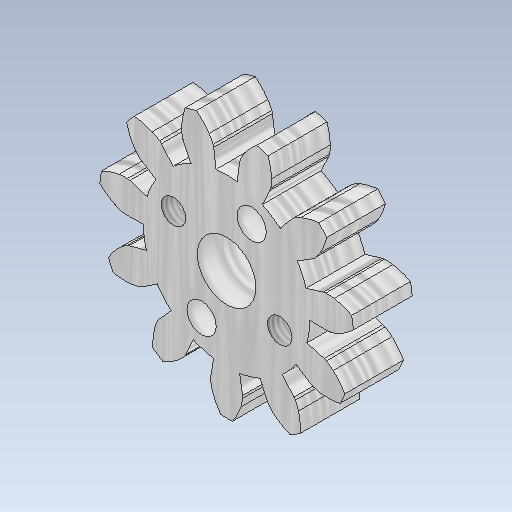
# Autodesk Inventor part: ｍ2歯数11ギア6td6
Saved by Autodesk Inventor 2020.2 (Build 242310000, 310)
## iProperties
Created: 2020-02-29
Part Number: ｍ2歯数11ギア6td6
Material: アルミニウム 7075
Document SubType Name: Modeling
Designer: aoyam
Density: 2.81 g/cm^3
Appearance: サテン - ブラシ仕上げ 重厚
Mass: 5.22906 g
Surface Area: 18.0274 cm^2
Volume: 1.86088 cm^3
Author: aoyam
Autodesk Inventor part; units mm, degrees
ref_plane "YZ Plane" through (0, 0, 0) normal (1, 0, 0) x (0, 1, 0)
ref_plane "XZ Plane" through (0, 0, 0) normal (0, 1, 0) x (-1, 0, 0)
ref_plane "XY Plane" through (0, 0, 0) normal (0, 0, 1) x (1, 0, 0)
sketch "スケッチ1" plane through (0, 0, 0) normal (0, 0, 1) x (1, 0, 0)
  arc A0 (-0.8026, 11.5515) -> (-0.8708, 11.3096) centre (0.3876, 11.0851) ccw
  arc A1 (-0.4025, 12.3114) -> (-0.8026, 11.5515) centre (2.526, 10.2842) ccw
  arc A2 (0.8885, 13.6879) -> (-0.4025, 12.3114) centre (4.8143, 8.7121) ccw
  arc A3 (-3.5076, 11.3096) -> (-3.5759, 11.5515) centre (-4.7661, 11.0851) ccw
  arc A4 (-3.5759, 11.5515) -> (-3.976, 12.3114) centre (-6.9045, 10.2842) ccw
  arc A5 (-3.976, 12.3114) -> (-5.267, 13.6879) centre (-9.1928, 8.7121) ccw
  arc A6 (-1.1051, 9.488) -> (-3.2734, 9.488) centre (-2.1892, 1.0574) ccw
  arc A7 (-5.267, 13.6879) -> (-6.4286, 13.3468) centre (-2.1892, 1.0574) ccw
  line L0 (-1.1051, 9.488) -> (-0.8708, 11.3096)
  line L1 (-3.2734, 9.488) -> (-3.5076, 11.3096)
  arc A8 (-6.6962, 10.6353) -> (-6.6229, 10.3949) centre (-5.4428, 10.8864) ccw
  arc A9 (-5.8351, 8.7358) -> (-7.6592, 7.5635) centre (-2.1892, 1.0574) ccw
  line L2 (-5.8351, 8.7358) -> (-6.6229, 10.3949)
  arc A10 (-6.7705, 11.4908) -> (-6.6962, 10.6353) centre (-3.2109, 11.3688) ccw
  arc A11 (-6.4286, 13.3468) -> (-6.7705, 11.4908) centre (-0.4359, 11.2834) ccw
  line L3 (-7.6592, 7.5635) -> (-8.8411, 8.9693)
  arc A12 (-8.8411, 8.9693) -> (-9.0293, 9.1359) centre (-9.7784, 8.1001) ccw
  arc A13 (-9.0293, 9.1359) -> (-9.7767, 9.5589) centre (-11.1444, 6.2702) ccw
  arc A14 (-11.6069, 10.0189) -> (-12.3997, 9.1039) centre (-2.1892, 1.0574) ccw
  arc A15 (-9.7767, 9.5589) -> (-11.6069, 10.0189) centre (-12.2195, 3.7106) ccw
  arc A16 (-11.159, 6.6782) -> (-10.9673, 6.5156) centre (-10.2402, 7.5671) ccw
  arc A17 (-9.4076, 5.5458) -> (-10.3083, 3.5734) centre (-2.1892, 1.0574) ccw
  line L4 (-9.4076, 5.5458) -> (-10.9673, 6.5156)
  arc A18 (-11.6839, 7.3577) -> (-11.159, 6.6782) centre (-8.6234, 9.1796) ccw
  arc A19 (-12.3997, 9.1039) -> (-11.6839, 7.3577) centre (-6.2428, 10.608) ccw
  line L5 (-10.3083, 3.5734) -> (-12.0626, 4.1171)
  arc A20 (-12.0626, 4.1171) -> (-12.311, 4.1555) centre (-12.3812, 2.8791) ccw
  arc A21 (-12.311, 4.1555) -> (-13.1684, 4.1072) centre (-12.541, 0.6012) ccw
  arc A22 (-14.9568, 3.5047) -> (-15.1291, 2.3063) centre (-2.1892, 1.0574) ccw
  arc A23 (-13.1684, 4.1072) -> (-14.9568, 3.5047) centre (-12.0616, -2.1334) ccw
  arc A24 (-12.7739, 0.9365) -> (-12.5247, 0.9034) centre (-12.4816, 2.181) ccw
  arc A25 (-10.6883, 0.9307) -> (-10.3797, -1.2155) centre (-2.1892, 1.0574) ccw
  line L6 (-10.6883, 0.9307) -> (-12.5247, 0.9034)
  arc A26 (-13.5829, 1.2244) -> (-12.7739, 0.9365) centre (-11.9932, 4.4116) ccw
  arc A27 (-15.1291, 2.3063) -> (-13.5829, 1.2244) centre (-10.7627, 6.9003) ccw
  line L7 (-10.3797, -1.2155) -> (-12.1494, -1.7066)
  arc A28 (-12.1494, -1.7066) -> (-12.3792, -1.8086) centre (-11.7481, -2.9203) ccw
  arc A29 (-12.3792, -1.8086) -> (-13.0744, -2.3127) centre (-10.6511, -4.923) ccw
  arc A30 (-14.2531, -3.7865) -> (-13.7502, -4.8877) centre (-2.1892, 1.0574) ccw
  arc A31 (-13.0744, -2.3127) -> (-14.2531, -3.7865) centre (-8.7693, -6.9642) ccw
  arc A32 (-11.0282, -4.7668) -> (-10.8007, -4.6599) centre (-11.4551, -3.5618) ccw
  arc A33 (-9.2706, -3.6441) -> (-7.8507, -5.2828) centre (-2.1892, 1.0574) ccw
  line L8 (-9.2706, -3.6441) -> (-10.8007, -4.6599)
  arc A34 (-11.8645, -4.962) -> (-11.0282, -4.7668) centre (-12.2502, -1.4213) ccw
  arc A35 (-13.7502, -4.8877) -> (-11.8645, -4.962) centre (-12.5606, 1.3376) ccw
  line L9 (-7.8507, -5.2828) -> (-9.074, -6.6527)
  arc A36 (-9.074, -6.6527) -> (-9.2121, -6.8627) centre (-8.0801, -7.4568) ccw
  arc A37 (-9.2121, -6.8627) -> (-9.5243, -7.6627) centre (-6.0745, -8.5484) ccw
  arc A38 (-9.7192, -9.5397) -> (-8.7007, -10.1943) centre (-2.1892, 1.0574) ccw
  arc A39 (-9.5243, -7.6627) -> (-9.7192, -9.5397) centre (-3.3879, -9.2483) ccw
  arc A40 (-6.4763, -8.6209) -> (-6.3426, -8.408) centre (-7.4868, -7.8381) ccw
  arc A41 (-5.6046, -6.7262) -> (-3.5242, -7.3371) centre (-2.1892, 1.0574) ccw
  line L10 (-5.6046, -6.7262) -> (-6.3426, -8.408)
  arc A42 (-7.0742, -9.2373) -> (-6.4763, -8.6209) centre (-9.313, -6.4672) ccw
  arc A43 (-8.7007, -10.1943) -> (-7.0742, -9.2373) centre (-11.0657, -4.3141) ccw
  line L11 (-3.5242, -7.3371) -> (-3.8126, -9.1509)
  arc A44 (-3.8126, -9.1509) -> (-3.8153, -9.4022) centre (-2.5419, -9.29) ccw
  arc A45 (-3.8153, -9.4022) -> (-3.6455, -10.244) centre (-0.2644, -9.1241) ccw
  arc A46 (-2.7946, -11.9285) -> (-1.5839, -11.9285) centre (-2.1892, 1.0574) ccw
  arc A47 (-3.6455, -10.244) -> (-2.7946, -11.9285) centre (2.3741, -8.2603) ccw
  arc A48 (-0.5632, -9.4022) -> (-0.5659, -9.1509) centre (-1.8366, -9.29) ccw
  arc A49 (-0.8543, -7.3371) -> (1.2262, -6.7262) centre (-2.1892, 1.0574) ccw
  line L12 (-0.8543, -7.3371) -> (-0.5659, -9.1509)
  arc A50 (-0.733, -10.244) -> (-0.5632, -9.4022) centre (-4.114, -9.1241) ccw
  arc A51 (-1.5839, -11.9285) -> (-0.733, -10.244) centre (-6.7525, -8.2603) ccw
  line L13 (1.2262, -6.7262) -> (1.9641, -8.408)
  arc A52 (1.9641, -8.408) -> (2.0978, -8.6209) centre (3.1084, -7.8381) ccw
  arc A53 (2.0978, -8.6209) -> (2.6957, -9.2373) centre (4.9345, -6.4672) ccw
  arc A54 (4.3222, -10.1943) -> (5.3407, -9.5397) centre (-2.1892, 1.0574) ccw
  arc A55 (2.6957, -9.2373) -> (4.3222, -10.1943) centre (6.6872, -4.3141) ccw
  arc A56 (4.8336, -6.8627) -> (4.6955, -6.6527) centre (3.7017, -7.4568) ccw
  arc A57 (3.4722, -5.2828) -> (4.8921, -3.6441) centre (-2.1892, 1.0574) ccw
  line L14 (3.4722, -5.2828) -> (4.6955, -6.6527)
  arc A58 (5.1459, -7.6627) -> (4.8336, -6.8627) centre (1.6961, -8.5484) ccw
  arc A59 (5.3407, -9.5397) -> (5.1459, -7.6627) centre (-0.9906, -9.2483) ccw
  line L15 (4.8921, -3.6441) -> (6.4222, -4.6599)
  arc A60 (6.4222, -4.6599) -> (6.6497, -4.7668) centre (7.0767, -3.5618) ccw
  arc A61 (6.6497, -4.7668) -> (7.486, -4.962) centre (7.8718, -1.4213) ccw
  arc A62 (9.3717, -4.8877) -> (9.8746, -3.7865) centre (-2.1892, 1.0574) ccw
  arc A63 (7.486, -4.962) -> (9.3717, -4.8877) centre (8.1822, 1.3376) ccw
  arc A64 (8.0007, -1.8086) -> (7.771, -1.7066) centre (7.3696, -2.9203) ccw
  arc A65 (6.0012, -1.2155) -> (6.3098, 0.9307) centre (-2.1892, 1.0574) ccw
  line L16 (6.0012, -1.2155) -> (7.771, -1.7066)
  arc A66 (8.6959, -2.3127) -> (8.0007, -1.8086) centre (6.2726, -4.923) ccw
  arc A67 (9.8746, -3.7865) -> (8.6959, -2.3127) centre (4.3908, -6.9642) ccw
  line L17 (6.3098, 0.9307) -> (8.1462, 0.9034)
  arc A68 (8.1462, 0.9034) -> (8.3954, 0.9365) centre (8.1031, 2.181) ccw
  arc A69 (8.3954, 0.9365) -> (9.2044, 1.2244) centre (7.6147, 4.4116) ccw
  arc A70 (10.7506, 2.3063) -> (10.5783, 3.5047) centre (-2.1892, 1.0574) ccw
  arc A71 (9.2044, 1.2244) -> (10.7506, 2.3063) centre (6.3843, 6.9003) ccw
  arc A72 (7.9326, 4.1555) -> (7.6842, 4.1171) centre (8.0027, 2.8791) ccw
  arc A73 (5.9299, 3.5734) -> (5.0291, 5.5458) centre (-2.1892, 1.0574) ccw
  line L18 (5.9299, 3.5734) -> (7.6842, 4.1171)
  arc A74 (8.7899, 4.1072) -> (7.9326, 4.1555) centre (8.1626, 0.6012) ccw
  arc A75 (10.5783, 3.5047) -> (8.7899, 4.1072) centre (7.6831, -2.1334) ccw
  line L19 (5.0291, 5.5458) -> (6.5888, 6.5156)
  arc A76 (6.5888, 6.5156) -> (6.7805, 6.6782) centre (5.8618, 7.5671) ccw
  arc A77 (6.7805, 6.6782) -> (7.3055, 7.3577) centre (4.245, 9.1796) ccw
  arc A78 (8.0213, 9.1039) -> (7.2284, 10.0189) centre (-2.1892, 1.0574) ccw
  arc A79 (7.3055, 7.3577) -> (8.0213, 9.1039) centre (1.8643, 10.608) ccw
  arc A80 (4.6508, 9.1359) -> (4.4626, 8.9693) centre (5.3999, 8.1001) ccw
  arc A81 (3.2807, 7.5635) -> (1.4566, 8.7358) centre (-2.1892, 1.0574) ccw
  line L20 (3.2807, 7.5635) -> (4.4626, 8.9693)
  arc A82 (5.3982, 9.5589) -> (4.6508, 9.1359) centre (6.7659, 6.2702) ccw
  arc A83 (7.2284, 10.0189) -> (5.3982, 9.5589) centre (7.841, 3.7106) ccw
  line L21 (1.4566, 8.7358) -> (2.2444, 10.3949)
  arc A84 (2.2444, 10.3949) -> (2.3178, 10.6353) centre (1.0643, 10.8864) ccw
  arc A85 (2.3178, 10.6353) -> (2.392, 11.4908) centre (-1.1676, 11.3688) ccw
  arc A86 (2.0501, 13.3468) -> (0.8885, 13.6879) centre (-2.1892, 1.0574) ccw
  arc A87 (2.392, 11.4908) -> (2.0501, 13.3468) centre (-3.9426, 11.2834) ccw
  circle A88 centre (-2.1892, 1.0574) radius 2.99
  circle A89 centre (0.3669, 6.4857) radius 1.495
  circle A90 centre (-2.1892, 1.0574) radius 8.5
  circle A91 centre (-4.7454, -4.3708) radius 1.495
  circle A92 centre (-7.6175, 3.6136) radius 1.25
  line L22 (-7.6175, 3.6136) -> (-2.1892, 1.0574)
  line L23 (0.3669, 6.4857) -> (-2.1892, 1.0574)
  circle A93 centre (3.239, -1.4987) radius 1.25
  point P0 (0, 0)
  point P1 (6.7805, 6.6782)
  point P2 (7.3055, 7.3577)
  point P3 (8.0213, 9.1039)
  point P4 (7.2284, 10.0189)
  point P5 (5.3982, 9.5589)
  point P6 (4.6508, 9.1359)
  point P7 (4.4626, 8.9693)
  point P8 (2.3178, 10.6353)
  point P9 (2.392, 11.4908)
  point P10 (2.0501, 13.3468)
  point P11 (0.8885, 13.6879)
  point P12 (-0.4025, 12.3114)
  point P13 (-0.8026, 11.5515)
  point P14 (-1.1051, 9.488)
  point P15 (-3.5759, 11.5515)
  point P16 (-3.976, 12.3114)
  point P17 (-5.267, 13.6879)
  point P18 (-6.4286, 13.3468)
  point P19 (-6.7705, 11.4908)
  point P20 (-6.6962, 10.6353)
  point P21 (-6.6229, 10.3949)
  point P22 (-5.8351, 8.7358)
  point P23 (-7.6592, 7.5635)
  point P24 (-9.0293, 9.1359)
  point P25 (-9.7767, 9.5589)
  point P26 (-11.6069, 10.0189)
  point P27 (-12.3997, 9.1039)
  point P28 (-11.6839, 7.3577)
  point P29 (-11.159, 6.6782)
  point P30 (-10.9673, 6.5156)
  point P31 (-12.311, 4.1555)
  point P32 (-13.1684, 4.1072)
  point P33 (-14.9568, 3.5047)
  point P34 (-15.1291, 2.3063)
  point P35 (-13.5829, 1.2244)
  point P36 (-12.7739, 0.9365)
  point P37 (-10.6883, 0.9307)
  point P38 (-10.3797, -1.2155)
  point P39 (-12.1494, -1.7066)
  point P40 (-12.3792, -1.8086)
  point P41 (-13.0744, -2.3127)
  point P42 (-14.2531, -3.7865)
  point P43 (-13.7502, -4.8877)
  point P44 (-11.8645, -4.962)
  point P45 (-11.0282, -4.7668)
  point P46 (-9.2706, -3.6441)
  point P47 (-9.2121, -6.8627)
  point P48 (-9.5243, -7.6627)
  point P49 (-9.7192, -9.5397)
  point P50 (-8.7007, -10.1943)
  point P51 (-7.0742, -9.2373)
  point P52 (-6.4763, -8.6209)
  point P53 (-3.8153, -9.4022)
  point P54 (-3.6455, -10.244)
  point P55 (-2.7946, -11.9285)
  point P56 (-1.5839, -11.9285)
  point P57 (-0.733, -10.244)
  point P58 (-0.5632, -9.4022)
  point P59 (-0.5659, -9.1509)
  point P60 (-0.8543, -7.3371)
  point P61 (2.0978, -8.6209)
  point P62 (2.6957, -9.2373)
  point P63 (4.3222, -10.1943)
  point P64 (5.3407, -9.5397)
  point P65 (5.1459, -7.6627)
  point P66 (4.8336, -6.8627)
  point P67 (4.6955, -6.6527)
  point P68 (6.6497, -4.7668)
  point P69 (7.486, -4.962)
  point P70 (9.3717, -4.8877)
  point P71 (9.8746, -3.7865)
  point P72 (8.6959, -2.3127)
  point P73 (8.0007, -1.8086)
  point P74 (7.771, -1.7066)
  point P75 (6.0012, -1.2155)
  point P76 (8.3954, 0.9365)
  point P77 (9.2044, 1.2244)
  point P78 (10.7506, 2.3063)
  point P79 (10.5783, 3.5047)
  point P80 (8.7899, 4.1072)
  point P81 (7.9326, 4.1555)
  dimension "d2" = 360
  dimension "d4" = 5.98
  dimension "d5" = 2.99
  dimension "d6" = 6
  dimension "d16" = 360
  dimension "d18" = 2.5
  dimension "d19" = 6
  dimension "d20" = 90
  dimension "d23" = 360
  constraints: 176 point on circle, 94 centre point, 48 end point, 4 coincident, 2 concentric, 429 other
  measures "d4" diameter of A88
  measures "d5" diameter of A89
  measures "d6" distance of A6.centre L23.start
  measures "d18" diameter of A92
  measures "d19" distance of L22.start A6.centre
  measures "d20" angle of L23 L22
extrude "押し出し1" add sketch "スケッチ1" along normal blind 6
thread "ねじ1" size "M3x0.5" class "6H" standard "ANSI Metric M Profile" full length
thread "ねじ2" size "M3x0.5" class "6H" standard "ANSI Metric M Profile" full length
